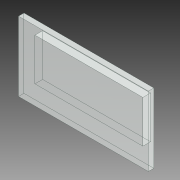
# Autodesk Inventor part: WindowInsert
Saved by Autodesk Inventor 2020 (Build 240168000, 168)
## iProperties
Created: 2020-08-04
Part Number: WindowInsert
Material: Glass
Document SubType Name: Modeling
Designer: DDeGo
Density: 2.18 g/cm^3
Appearance: Clear
Author: DDeGo
Autodesk Inventor part; units mm, degrees
ref_plane "YZ Plane" through (0, 0, 0) normal (1, 0, 0) x (0, 1, 0)
ref_plane "XZ Plane" through (0, 0, 0) normal (0, 1, 0) x (-1, 0, 0)
ref_plane "XY Plane" through (0, 0, 0) normal (0, 0, 1) x (1, 0, 0)
sketch "Sketch1" plane through (0, 0, 0) normal (0, 0, 1) x (1, 0, 0)
  line L0 (-9.85, -3.85) -> (9.85, -3.85)
  line L1 (9.85, -3.85) -> (9.85, 3.85)
  line L2 (9.85, 3.85) -> (-9.85, 3.85)
  line L3 (-9.85, 3.85) -> (-9.85, -3.85)
  line L4 (-9.85, -3.85) -> (9.85, 3.85) construction
  line L5 (9.85, -3.85) -> (-9.85, 3.85) construction
  point P0 (0, 0)
  dimension "d0" = 19.7
  dimension "d1" = 7.7
  constraints: 12 end point, 2 midpoint, 2 parallel, 1 horizontal, 1 perpendicular
  measures "d0" distance of L1.end L2.end
  measures "d1" distance of L0.end L1.end
extrude "Extrusion1" add sketch "Sketch1" along normal blind 1.4
sketch "Sketch2" plane through (0, 0, 1.4) normal (0, 0, 1) x (1, 0, 0)
  line L0 (-11.85, -6.35) -> (11.85, -6.35)
  line L1 (11.85, -6.35) -> (11.85, 6.35)
  line L2 (11.85, 6.35) -> (-11.85, 6.35)
  line L3 (-11.85, 6.35) -> (-11.85, -6.35)
  line L4 (-11.85, -6.35) -> (11.85, 6.35) construction
  line L5 (11.85, -6.35) -> (-11.85, 6.35) construction
  point P0 (0, 0)
  dimension "d4" = 23.7
  dimension "d5" = 12.7
  constraints: 12 end point, 2 midpoint, 2 parallel, 1 horizontal, 1 perpendicular
  measures "d4" distance of L1.end L2.end
  measures "d5" distance of L0.end L1.end
extrude "Extrusion2" add sketch "Sketch2" along normal blind 1
body "Solid1"
